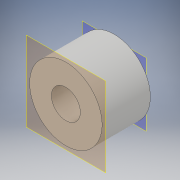
# Autodesk Inventor part: spannring_achse
Saved by Autodesk Inventor 2017 (Build 210142000, 142)
## iProperties
Part Number: spannring_achse
Material: Generisch
Document SubType Name: Modeling
Designer: Fabio
Density: 1 g/cm^3
Appearance: Vorgabe
Author: Fabio
Autodesk Inventor part; units mm, degrees
ref_plane "YZ Plane" through (0, 0, 0) normal (1, 0, 0) x (0, 1, 0)
ref_plane "XZ Plane" through (0, 0, 0) normal (0, 1, 0) x (-1, 0, 0)
ref_plane "XY Plane" through (0, 0, 0) normal (0, 0, 1) x (1, 0, 0)
sketch "Skizze1" plane through (0, 0, 0) normal (0, 1, 0) x (-1, 0, 0)
  circle A0 centre (0, 0) radius 7.5
  dimension "d0" = 15
  constraints: 1 centre point, 1 coincident
  measures "d0" diameter of A0
extrude "Extrusion1" add sketch "Skizze1" along normal blind 10
ref_plane "Arbeitsebene1" through (0, 10, 0) normal (0, 1, 0) x (1, 0, 0)
sketch "Skizze2" plane through (0, 10, 0) normal (0, 1, 0) x (1, 0, 0)
  circle A0 centre (0, 0) radius 7.5 projected
  circle A1 centre (0, 0) radius 7.5 construction
  circle A2 centre (0, 0) radius 7.5 construction
  line L0 (0, 0) -> (0, 5) construction
  line L1 (0, 0) -> (0, -5) construction
  dimension "d4" = 5
  dimension "d5" = 5
  constraints: 4 end point, 2 vertical
  measures "d4" distance of point (0, 0) L1.end
  measures "d5" distance of L0.end point (0, 0)
hole "Bohrung1" at (0, 10, 5) at (0, 10, -5) direction (0, -1, 0) diameter 3 depth 5 tip angle 118
thread "Gewinde1" size "M3x0.5" class "6H" standard "ANSI Metric M Profile" full length
thread "Gewinde2" size "M3x0.5" class "6H" standard "ANSI Metric M Profile" full length
ref_plane "Arbeitsebene2" through (0, 0, 0) normal (0, -1, 0) x (1, 0, 0)
sketch "Skizze3" plane through (0, 0, 0) normal (0, -1, 0) x (1, 0, 0)
  circle A0 centre (0, 0) radius 7.5 projected
  constraints: 1 coincident
hole "Bohrung2" at (0, 0, 0) direction (0, 1, 0) diameter 6 end through all
